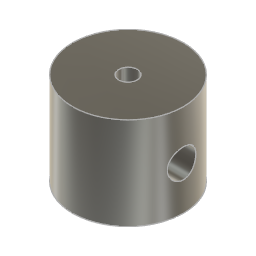
coupling gear v2 v2 (Autodesk Fusion 360 design; units mm, degrees)
Autodesk Fusion 360 part; units mm, degrees
sketch "Sketch1" plane through (0, 0, 0) normal (0, 0, 1) x (1, 0, 0)
  circle A0 centre (0, 0) radius 6
  circle A1 centre (0, 0) radius 1
  dimension "d1" = 2
  dimension "d12" = 12
  constraint coincident A0.centre A1.centre
  measures "d1" diameter of A1
  measures "d12" diameter of A0
extrude "Extrude1" add sketch "Sketch1" along normal blind 10
sketch "Sketch2" plane through (0, 0, 0) normal (1, 0, 0) x (0, 1, 0)
  circle A0 centre (0, 4.686) radius 1.55
  dimension "d4" = 3.1
  measures "d4" diameter of A0
extrude "Extrude2" cut sketch "Sketch2" along normal blind 12
sketch "Sketch3" plane through (0, 0, 10) normal (0, 0, 1) x (-1, 0, 0)
  circle A0 centre (0, 0) radius 1
  circle A1 centre (0, 0) radius 6
  line L0 (-2, 0.003) -> (-2, 3.003)
  line L1 (-2, 0.003) -> (-2, -2.997)
  line L2 (-2, 3.003) -> (-4.5, 3.003)
  line L3 (-2, -2.997) -> (-4.5, -2.997)
  line L4 (-4.5, 3.003) -> (-4.5, -2.997)
  dimension "d7" = 3
  dimension "d8" = 3
  dimension "d9" = 2.5
  dimension "d10" = 2.5
  dimension "d11" = 2
  constraint vertical L0
  constraint parallel L0 L1
  constraint perpendicular L0 L2
  constraint perpendicular L1 L3
  measures "d7" distance of L0.start L0.end
  measures "d8" distance of L0.start L1.end
  measures "d9" distance of L0.end L2.end
  measures "d10" distance of L1.end L3.end
  measures "d11" distance of A0.centre L0
extrude "Extrude3" [suppressed]
